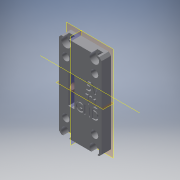
# Autodesk Inventor part: 02_Camera_Lid
Saved by Autodesk Inventor 2019.4 (Build 234330000, 330)
## iProperties
Created: 2021-09-23
Part Number: 02_Camera_Lid
Material: Generisch
Document SubType Name: Modeling
Designer: Muriel
Density: 1 g/cm^3
Appearance: Vorgabe
Author: Muriel
Autodesk Inventor part; units mm, degrees
ref_plane "YZ Plane" through (0, 0, 0) normal (1, 0, 0) x (0, 1, 0)
ref_plane "XZ Plane" through (0, 0, 0) normal (0, 1, 0) x (-1, 0, 0)
ref_plane "XY Plane" through (0, 0, 0) normal (0, 0, 1) x (1, 0, 0)
ref_plane "Arbeitsebene1" through (0, 0, 0) normal (0, 0, 1) x (1, 0, 0)
sketch "Skizze1" plane through (0, 0, 0) normal (0, 0, 1) x (1, 0, 0)
  line L0 (-3.05, 28.45) -> (-3.05, 27.95) projected
  line L1 (-2.75, 27.95) -> (-3.05, 27.95) projected
  line L2 (-1.75, 26.95) -> (-2.75, 27.95) projected
  line L3 (-1.75, 26.25) -> (-1.75, 26.95) projected
  line L4 (1.1, 26.25) -> (-1.75, 26.25) projected
  line L5 (1.1, 0.85) -> (1.1, 26.25) projected
  line L6 (1.1, 0.85) -> (-1.75, 0.85) projected
  line L7 (-1.75, 0.85) -> (-1.75, 0.15) projected
  line L8 (-2.75, -0.85) -> (-1.75, 0.15) projected
  line L9 (-2.75, -0.85) -> (-3.05, -0.85) projected
  line L10 (-3.05, -0.85) -> (-3.05, -1.35) projected
  line L11 (-3.05, -1.35) -> (-12.95, -1.35) projected
  line L12 (-12.95, -1.35) -> (-12.95, -0.35) projected
  line L13 (-12.95, -0.35) -> (-13.95, -0.35) projected
  line L14 (-13.95, -0.35) -> (-13.95, -1.35) projected
  line L15 (-13.95, -1.35) -> (-15.2198, -1.35) projected
  line L16 (-15.2198, -1.35) -> (-15.2198, 0.65) projected
  line L17 (-15.2198, 0.65) -> (-16.05, 0.65) projected
  line L18 (-16.05, 0.65) -> (-16.05, -3.35) projected
  line L19 (-15.05, -4.35) -> (-16.05, -3.35) projected
  line L20 (-15.05, -4.35) -> (0.75, -4.35) projected
  line L21 (1.75, -3.35) -> (0.75, -4.35) projected
  line L22 (1.75, -3.35) -> (1.75, 30.45) projected
  line L23 (0.75, 31.45) -> (1.75, 30.45) projected
  line L24 (-15.05, 31.45) -> (0.75, 31.45) projected
  line L25 (-16.05, 30.45) -> (-15.05, 31.45) projected
  line L26 (-16.05, 26.45) -> (-16.05, 30.45) projected
  line L27 (-16.05, 26.45) -> (-15.2198, 26.45) projected
  line L28 (-15.2198, 26.45) -> (-15.2198, 28.45) projected
  line L29 (-15.2198, 28.45) -> (-13.95, 28.45) projected
  line L30 (-13.95, 28.45) -> (-13.95, 27.45) projected
  line L31 (-13.95, 27.45) -> (-12.95, 27.45) projected
  line L32 (-12.95, 27.45) -> (-12.95, 28.45) projected
  line L33 (-12.95, 28.45) -> (-3.05, 28.45) projected
  circle A0 centre (-1.25, 29.85) radius 0.95 projected
  circle A1 centre (-13.05, 29.85) radius 0.95 projected
  circle A2 centre (-13.05, -2.75) radius 0.95 projected
  circle A3 centre (-1.25, -2.75) radius 0.95 projected
  line L34 (-16.05, 26.45) -> (-16.05, 0.65)
  point P0 (0, 0)
  constraints: 2 end point, 1 vertical
extrude "Extrusion1" add sketch "Skizze1" along normal blind 4
sketch "Skizze2" plane through (0, 0, 4) normal (0, 0, 1) x (1, 0, 0)
  circle A0 centre (-1.25, -2.75) radius 0.95 projected
  circle A1 centre (-13.05, -2.75) radius 0.95 projected
  circle A2 centre (-13.05, 29.85) radius 0.95 projected
  circle A3 centre (-1.25, 29.85) radius 0.95 projected
  line L0 (-16.05, 30.45) -> (-16.05, -3.35) projected
  line L1 (-16.05, -3.35) -> (-15.05, -4.35) projected
  line L2 (-15.05, -4.35) -> (0.75, -4.35) projected
  line L3 (0.75, -4.35) -> (1.75, -3.35) projected
  line L4 (1.75, -3.35) -> (1.75, 30.45) projected
  line L5 (1.75, 30.45) -> (0.75, 31.45) projected
  line L6 (0.75, 31.45) -> (-15.05, 31.45) projected
  line L7 (-15.05, 31.45) -> (-16.05, 30.45) projected
  point P0 (0, 0)
hole "Bohrung1" at (-1.25, 29.85, 4) at (-13.05, 29.85, 4) at (-1.25, -2.75, 4) at (-13.05, -2.75, 4) direction (0, 0, -1) diameter 2 depth 12 tip angle 118 counterbore diameter 4 counterbore depth 2.5
sketch "Skizze5" plane through (0, 0, 4) normal (0, 0, 1) x (1, 0, 0)
  line L0 (-5.0417, 20.4942) -> (0.4976, 20.4942) construction
  line L1 (0.4976, 20.4942) -> (0.4976, 16.9204) construction
  line L2 (0.4976, 16.9204) -> (-5.0417, 16.9204) construction
  line L3 (-5.0417, 16.9204) -> (-5.0417, 20.4942) construction
  line L4 (-9.0877, 11.2435) -> (0.5466, 11.2435) construction
  line L5 (0.5466, 11.2435) -> (0.5466, 7.613) construction
  line L6 (0.5466, 7.613) -> (-9.0877, 7.613) construction
  line L7 (-9.0877, 7.613) -> (-9.0877, 11.2435) construction
  line L8 (-5.1084, 15.6437) -> (0.3288, 15.6437) construction
  line L9 (0.3288, 15.6437) -> (0.3288, 12.1323) construction
  line L10 (0.3288, 12.1323) -> (-5.1084, 12.1323) construction
  line L11 (-5.1084, 12.1323) -> (-5.1084, 15.6437) construction
  spline S0 degree 2 poles (-2.6649, 18.106) (-2.6649, 17.8536) (-2.8266, 17.4225) (-2.9741, 17.2636) knots 0 0 0 1 2 2 2
  spline S1 degree 2 poles (-2.9741, 17.2636) (-3.1216, 17.1048) (-3.5612, 16.9204) (-3.8335, 16.9204) knots 0 0 0 1 2 2 2
  spline S2 degree 2 poles (-3.8335, 16.9204) (-4.0831, 16.9204) (-4.5709, 17.0311) (-4.7496, 17.119) knots 0 0 0 1 2 2 2
  line L12 (-4.7496, 17.119) -> (-4.7496, 17.6153)
  line L13 (-4.7496, 17.6153) -> (-4.7156, 17.6153)
  spline S3 degree 2 poles (-4.7156, 17.6153) (-4.6617, 17.5756) (-4.4603, 17.4735) (-4.3383, 17.4281) knots 0 0 0 1 2 2 2
  spline S4 degree 2 poles (-4.3383, 17.4281) (-4.1994, 17.3799) (-3.9696, 17.326) (-3.825, 17.326) knots 0 0 0 1 2 2 2
  spline S5 degree 2 poles (-3.825, 17.326) (-3.6831, 17.326) (-3.4165, 17.4281) (-3.3201, 17.5388) knots 0 0 0 1 2 2 2
  spline S6 degree 2 poles (-3.3201, 17.5388) (-3.2322, 17.6437) (-3.1414, 17.9217) (-3.1414, 18.1089) knots 0 0 0 1 2 2 2
  spline S7 degree 2 poles (-3.1414, 18.1089) (-3.1414, 18.2961) (-3.2435, 18.5343) (-3.34, 18.6137) knots 0 0 0 1 2 2 2
  spline S8 degree 2 poles (-3.34, 18.6137) (-3.4392, 18.7016) (-3.7342, 18.7754) (-3.9129, 18.7754) knots 0 0 0 1 2 2 2
  spline S9 degree 2 poles (-3.9129, 18.7754) (-4.1058, 18.7754) (-4.4887, 18.7158) (-4.6049, 18.6903) knots 0 0 0 1 2 2 2
  line L14 (-4.6049, 18.6903) -> (-4.6049, 20.4942)
  line L15 (-4.6049, 20.4942) -> (-2.6848, 20.4942)
  line L16 (-2.6848, 20.4942) -> (-2.6848, 20.0829)
  line L17 (-2.6848, 20.0829) -> (-4.154, 20.0829)
  line L18 (-4.154, 20.0829) -> (-4.154, 19.1498)
  spline S10 degree 2 poles (-4.154, 19.1498) (-4.0689, 19.1611) (-3.9044, 19.1696) (-3.8363, 19.1696) knots 0 0 0 1 2 2 2
  spline S11 degree 2 poles (-3.8363, 19.1696) (-3.5669, 19.1696) (-3.1953, 19.0817) (-3.0251, 18.9512) knots 0 0 0 1 2 2 2
  spline S12 degree 2 poles (-3.0251, 18.9512) (-2.8521, 18.8208) (-2.6649, 18.4237) (-2.6649, 18.106) knots 0 0 0 1 2 2 2
  line L19 (0.4777, 20.4942) -> (-0.7277, 16.9942)
  line L20 (-0.7277, 16.9942) -> (-1.2297, 16.9942)
  line L21 (-1.2297, 16.9942) -> (-2.4352, 20.4942)
  line L22 (-2.4352, 20.4942) -> (-1.936, 20.4942)
  line L23 (-1.936, 20.4942) -> (-0.966, 17.587)
  line L24 (-0.966, 17.587) -> (0.004, 20.4942)
  line L25 (0.004, 20.4942) -> (0.4777, 20.4942)
  line L26 (-3.937, 12.1323) -> (-3.937, 15.2182)
  line L27 (-3.937, 15.2182) -> (-5.1113, 15.2182)
  line L28 (-5.1113, 15.2182) -> (-5.1113, 15.6323)
  line L29 (-5.1113, 15.6323) -> (-2.2976, 15.6323)
  line L30 (-2.2976, 15.6323) -> (-2.2976, 15.2182)
  line L31 (-2.2976, 15.2182) -> (-3.4719, 15.2182)
  line L32 (-3.4719, 15.2182) -> (-3.4719, 12.1323)
  line L33 (-3.4719, 12.1323) -> (-3.937, 12.1323)
  line L34 (-0.0598, 12.1323) -> (-1.7673, 12.1323)
  line L35 (-1.7673, 12.1323) -> (-1.7673, 12.4897)
  line L36 (-1.7673, 12.4897) -> (-1.1319, 12.4897)
  line L37 (-1.1319, 12.4897) -> (-1.1319, 14.8353)
  line L38 (-1.1319, 14.8353) -> (-1.7673, 14.8353)
  line L39 (-1.7673, 14.8353) -> (-1.7673, 15.1558)
  spline S13 degree 2 poles (-1.7673, 15.1558) (-1.407, 15.1558) (-1.0667, 15.36) (-1.044, 15.6437) knots 0 0 0 1 2 2 2
  line L40 (-1.044, 15.6437) -> (-0.6809, 15.6437)
  line L41 (-0.6809, 15.6437) -> (-0.6809, 12.4897)
  line L42 (-0.6809, 12.4897) -> (-0.0598, 12.4897)
  line L43 (-0.0598, 12.4897) -> (-0.0598, 12.1323)
  spline S14 degree 2 poles (-7.2668, 7.613) (-7.6384, 7.613) (-8.2538, 7.8399) (-8.4751, 8.0696) knots 0 0 0 1 2 2 2
  spline S15 degree 2 poles (-8.4751, 8.0696) (-8.6963, 8.3022) (-8.9317, 8.9886) (-8.9317, 9.4339) knots 0 0 0 1 2 2 2
  spline S16 degree 2 poles (-8.9317, 9.4339) (-8.9317, 9.8565) (-8.6935, 10.5259) (-8.4722, 10.7641) knots 0 0 0 1 2 2 2
  spline S17 degree 2 poles (-8.4722, 10.7641) (-8.2595, 10.9939) (-7.6355, 11.2435) (-7.264, 11.2435) knots 0 0 0 1 2 2 2
  spline S18 degree 2 poles (-7.264, 11.2435) (-7.0853, 11.2435) (-6.7619, 11.1924) (-6.6144, 11.147) knots 0 0 0 1 2 2 2
  spline S19 degree 2 poles (-6.6144, 11.147) (-6.4953, 11.113) (-6.206, 10.9882) (-6.1181, 10.9428) knots 0 0 0 1 2 2 2
  line L44 (-6.1181, 10.9428) -> (-6.1181, 10.3812)
  line L45 (-6.1181, 10.3812) -> (-6.1578, 10.3812)
  spline S20 degree 2 poles (-6.1578, 10.3812) (-6.2457, 10.4578) (-6.4301, 10.5968) (-6.6003, 10.6762) knots 0 0 0 1 2 2 2
  spline S21 degree 2 poles (-6.6003, 10.6762) (-6.7421, 10.7471) (-7.108, 10.8407) (-7.3179, 10.8407) knots 0 0 0 1 2 2 2
  spline S22 degree 2 poles (-7.3179, 10.8407) (-7.8227, 10.8407) (-8.4467, 10.0806) (-8.4467, 9.4481) knots 0 0 0 1 2 2 2
  spline S23 degree 2 poles (-8.4467, 9.4481) (-8.4467, 9.0964) (-8.2822, 8.5688) (-8.1262, 8.3873) knots 0 0 0 1 2 2 2
  spline S24 degree 2 poles (-8.1262, 8.3873) (-7.9759, 8.2058) (-7.5504, 8.0157) (-7.2838, 8.0157) knots 0 0 0 1 2 2 2
  spline S25 degree 2 poles (-7.2838, 8.0157) (-7.0881, 8.0157) (-6.6967, 8.0725) (-6.5634, 8.1292) knots 0 0 0 1 2 2 2
  line L46 (-6.5634, 8.1292) -> (-6.5634, 9.034)
  line L47 (-6.5634, 9.034) -> (-7.3746, 9.034)
  line L48 (-7.3746, 9.034) -> (-7.3746, 9.4424)
  line L49 (-7.3746, 9.4424) -> (-6.1039, 9.4424)
  line L50 (-6.1039, 9.4424) -> (-6.1039, 7.9136)
  spline S26 degree 2 poles (-6.1039, 7.9136) (-6.1918, 7.8739) (-6.4925, 7.752) (-6.6201, 7.7151) knots 0 0 0 1 2 2 2
  spline S27 degree 2 poles (-6.6201, 7.7151) (-6.7931, 7.664) (-7.0711, 7.613) (-7.2668, 7.613) knots 0 0 0 1 2 2 2
  line L51 (-3.0152, 7.6811) -> (-3.5371, 7.6811)
  line L52 (-3.5371, 7.6811) -> (-5.0857, 10.6989)
  line L53 (-5.0857, 10.6989) -> (-5.0857, 7.6811)
  line L54 (-5.0857, 7.6811) -> (-5.5196, 7.6811)
  line L55 (-5.5196, 7.6811) -> (-5.5196, 11.1811)
  line L56 (-5.5196, 11.1811) -> (-4.8588, 11.1811)
  line L57 (-4.8588, 11.1811) -> (-3.4491, 8.41)
  line L58 (-3.4491, 8.41) -> (-3.4491, 11.1811)
  line L59 (-3.4491, 11.1811) -> (-3.0152, 11.1811)
  line L60 (-3.0152, 11.1811) -> (-3.0152, 7.6811)
  spline S28 degree 2 poles (0.4536, 9.4282) (0.4536, 8.9489) (0.065, 8.1774) (-0.2611, 7.9619) knots 0 0 0 1 2 2 2
  spline S29 degree 2 poles (-0.2611, 7.9619) (-0.5277, 7.7945) (-1.0751, 7.6811) (-1.5006, 7.6811) knots 0 0 0 1 2 2 2
  line L61 (-1.5006, 7.6811) -> (-2.3061, 7.6811)
  line L62 (-2.3061, 7.6811) -> (-2.3061, 11.1811)
  line L63 (-2.3061, 11.1811) -> (-1.5091, 11.1811)
  spline S30 degree 2 poles (-1.5091, 11.1811) (-1.0156, 11.1811) (-0.454, 11.0336) (-0.2555, 10.9031) knots 0 0 0 1 2 2 2
  spline S31 degree 2 poles (-0.2555, 10.9031) (0.0821, 10.679) (0.4536, 9.9388) (0.4536, 9.4282) knots 0 0 0 1 2 2 2
  spline S32 degree 2 poles (-0.0314, 9.4339) (-0.0314, 9.8367) (-0.298, 10.4068) (-0.5618, 10.5684) knots 0 0 0 1 2 2 2
  spline S33 degree 2 poles (-0.5618, 10.5684) (-0.749, 10.679) (-1.1716, 10.7783) (-1.4864, 10.7783) knots 0 0 0 1 2 2 2
  line L64 (-1.4864, 10.7783) -> (-1.8409, 10.7783)
  line L65 (-1.8409, 10.7783) -> (-1.8409, 8.0838)
  line L66 (-1.8409, 8.0838) -> (-1.4864, 8.0838)
  spline S34 degree 2 poles (-1.4864, 8.0838) (-1.1773, 8.0838) (-0.7093, 8.1831) (-0.5192, 8.3164) knots 0 0 0 1 2 2 2
  spline S35 degree 2 poles (-0.5192, 8.3164) (-0.2753, 8.4809) (-0.0314, 9.0255) (-0.0314, 9.4339) knots 0 0 0 1 2 2 2
  point P0 (0, 0)
  constraints: 6 other
extrude "Extrusion3" cut sketch "Skizze5" against normal blind 1
sketch "Skizze6" plane through (0, 0, 4) normal (0, 0, 1) x (1, 0, 0)
  arc A0 (-0.05, -4.35) -> (-2.45, -4.35) centre (-1.25, -2.75) ccw projected
  line L0 (-0.05, -4.35) -> (0.75, -4.35) projected
  line L1 (0.75, -4.35) -> (1.75, -3.35) projected
  line L2 (1.75, -3.35) -> (1.75, 30.45) projected
  line L3 (1.75, 30.45) -> (0.75, 31.45) projected
  line L4 (0.75, 31.45) -> (-0.05, 31.45) projected
  arc A1 (-2.45, 31.45) -> (-0.05, 31.45) centre (-1.25, 29.85) ccw projected
  line L5 (-2.45, 31.45) -> (-11.85, 31.45) projected
  arc A2 (-14.25, 31.45) -> (-11.85, 31.45) centre (-13.05, 29.85) ccw projected
  line L6 (-14.25, 31.45) -> (-15.05, 31.45) projected
  line L7 (-15.05, 31.45) -> (-16.05, 30.45) projected
  line L8 (-16.05, 30.45) -> (-16.05, -3.35) projected
  line L9 (-16.05, -3.35) -> (-15.05, -4.35) projected
  line L10 (-15.05, -4.35) -> (-14.25, -4.35) projected
  arc A3 (-11.85, -4.35) -> (-14.25, -4.35) centre (-13.05, -2.75) ccw projected
  line L11 (-11.85, -4.35) -> (-2.45, -4.35) projected
  line L12 (-3.0152, 11.1811) -> (-3.0152, 7.6811) projected
  line L13 (-3.0152, 7.6811) -> (-3.5371, 7.6811) projected
  line L14 (-3.5371, 7.6811) -> (-5.0857, 10.6989) projected
  line L15 (-5.0857, 10.6989) -> (-5.0857, 7.6811) projected
  line L16 (-5.0857, 7.6811) -> (-5.5196, 7.6811) projected
  line L17 (-5.5196, 7.6811) -> (-5.5196, 11.1811) projected
  line L18 (-5.5196, 11.1811) -> (-4.8588, 11.1811) projected
  line L19 (-4.8588, 11.1811) -> (-3.4491, 8.41) projected
  line L20 (-3.4491, 8.41) -> (-3.4491, 11.1811) projected
  line L21 (-3.4491, 11.1811) -> (-3.0152, 11.1811) projected
  line L22 (-0.0598, 12.4897) -> (-0.0598, 12.1323) projected
  line L23 (-0.0598, 12.1323) -> (-1.7673, 12.1323) projected
  line L24 (-1.7673, 12.1323) -> (-1.7673, 12.4897) projected
  line L25 (-1.7673, 12.4897) -> (-1.1319, 12.4897) projected
  line L26 (-1.1319, 12.4897) -> (-1.1319, 14.8353) projected
  line L27 (-1.1319, 14.8353) -> (-1.7673, 14.8353) projected
  line L28 (-1.7673, 14.8353) -> (-1.7673, 15.1558) projected
  line L29 (-1.044, 15.6437) -> (-0.6809, 15.6437) projected
  line L30 (-0.6809, 15.6437) -> (-0.6809, 12.4897) projected
  line L31 (-0.6809, 12.4897) -> (-0.0598, 12.4897) projected
  line L32 (0.004, 20.4942) -> (0.4777, 20.4942) projected
  line L33 (0.4777, 20.4942) -> (-0.7277, 16.9942) projected
  line L34 (-0.7277, 16.9942) -> (-1.2297, 16.9942) projected
  line L35 (-1.2297, 16.9942) -> (-2.4352, 20.4942) projected
  line L36 (-2.4352, 20.4942) -> (-1.936, 20.4942) projected
  line L37 (-1.936, 20.4942) -> (-0.966, 17.587) projected
  line L38 (-0.966, 17.587) -> (0.004, 20.4942) projected
  line L39 (-4.7496, 17.119) -> (-4.7496, 17.6153) projected
  line L40 (-4.7496, 17.6153) -> (-4.7156, 17.6153) projected
  line L41 (-4.6049, 18.6903) -> (-4.6049, 20.4942) projected
  line L42 (-4.6049, 20.4942) -> (-2.6848, 20.4942) projected
  line L43 (-2.6848, 20.4942) -> (-2.6848, 20.0829) projected
  line L44 (-2.6848, 20.0829) -> (-4.154, 20.0829) projected
  line L45 (-4.154, 20.0829) -> (-4.154, 19.1498) projected
  line L46 (-3.4719, 12.1323) -> (-3.937, 12.1323) projected
  line L47 (-3.937, 12.1323) -> (-3.937, 15.2182) projected
  line L48 (-3.937, 15.2182) -> (-5.1113, 15.2182) projected
  line L49 (-5.1113, 15.2182) -> (-5.1113, 15.6323) projected
  line L50 (-5.1113, 15.6323) -> (-2.2976, 15.6323) projected
  line L51 (-2.2976, 15.6323) -> (-2.2976, 15.2182) projected
  line L52 (-2.2976, 15.2182) -> (-3.4719, 15.2182) projected
  line L53 (-3.4719, 15.2182) -> (-3.4719, 12.1323) projected
  line L54 (-6.1181, 10.9428) -> (-6.1181, 10.3812) projected
  line L55 (-6.1181, 10.3812) -> (-6.1578, 10.3812) projected
  line L56 (-6.5634, 8.1292) -> (-6.5634, 9.034) projected
  line L57 (-6.5634, 9.034) -> (-7.3746, 9.034) projected
  line L58 (-7.3746, 9.034) -> (-7.3746, 9.4424) projected
  line L59 (-7.3746, 9.4424) -> (-6.1039, 9.4424) projected
  line L60 (-6.1039, 9.4424) -> (-6.1039, 7.9136) projected
  line L61 (-1.5006, 7.6811) -> (-2.3061, 7.6811) projected
  line L62 (-2.3061, 7.6811) -> (-2.3061, 11.1811) projected
  line L63 (-2.3061, 11.1811) -> (-1.5091, 11.1811) projected
  line L64 (-9.6163, 19.7) -> (-9.6163, 7.4)
  line L65 (-9.6163, 7.4) -> (-12.1163, 7.4)
  line L66 (-12.1163, 7.4) -> (-12.1163, 19.7)
  line L67 (-12.1163, 19.7) -> (-9.6163, 19.7)
  line L68 (-9.6163, 19.7) -> (-12.1163, 7.4) construction
  line L69 (-9.6163, 7.4) -> (-12.1163, 19.7) construction
  point P0 (0, 0)
  point P1 (-10.8663, 13.55)
  dimension "d31" = 12.3
  dimension "d32" = 2.5
  dimension "d38" = 17.9
  constraints: 12 end point, 2 midpoint, 2 parallel, 1 perpendicular, 1 vertical, 32 other
  measures "d31" distance of L64.start L64.end
  measures "d32" distance of L64.end L65.end
  measures "d38" distance from line of point (-10.866, 13.55) L11
extrude "Extrusion4" cut sketch "Skizze6" against normal blind 10 contours L64 L65 L66 L67
sketch "Skizze7" plane through (-16.05, -3.35, 0) normal (-1, 0, 0) x (0, 0, 1)
  line L0 (0, 33.8) -> (0, 0) projected
  line L1 (0, 0) -> (4, 0) projected
  line L2 (4, 33.8) -> (4, 0) projected
  line L3 (0, 33.8) -> (4, 33.8) projected
  circle A0 centre (2, 16.9) radius 1.4
  point P0 (0, 3.35)
  dimension "d35" = 2.8
  constraints: 1 centre point
  measures "d35" diameter of A0
extrude "Extrusion5" cut sketch "Skizze7" against normal up to next contours A0
sketch "Skizze8" plane through (0, 0, 4) normal (0, 0, 1) x (1, 0, 0)
  line L0 (-12.1163, 19.7) -> (-9.6163, 19.7) projected
  line L1 (-9.6163, 19.7) -> (-9.6163, 7.4) projected
  line L2 (-9.6163, 7.4) -> (-12.1163, 7.4) projected
  line L3 (-12.1163, 7.4) -> (-12.1163, 19.7) projected
  arc A0 (-0.05, -4.35) -> (-2.45, -4.35) centre (-1.25, -2.75) ccw projected
  line L4 (-0.05, -4.35) -> (0.75, -4.35) projected
  line L5 (0.75, -4.35) -> (1.75, -3.35) projected
  line L6 (1.75, -3.35) -> (1.75, 30.45) projected
  line L7 (1.75, 30.45) -> (0.75, 31.45) projected
  line L8 (0.75, 31.45) -> (-0.05, 31.45) projected
  arc A1 (-2.45, 31.45) -> (-0.05, 31.45) centre (-1.25, 29.85) ccw projected
  line L9 (-2.45, 31.45) -> (-11.85, 31.45) projected
  arc A2 (-14.25, 31.45) -> (-11.85, 31.45) centre (-13.05, 29.85) ccw projected
  line L10 (-14.25, 31.45) -> (-15.05, 31.45) projected
  line L11 (-15.05, 31.45) -> (-16.05, 30.45) projected
  line L12 (-16.05, 30.45) -> (-16.05, -3.35) projected
  line L13 (-16.05, -3.35) -> (-15.05, -4.35) projected
  line L14 (-15.05, -4.35) -> (-14.25, -4.35) projected
  arc A3 (-11.85, -4.35) -> (-14.25, -4.35) centre (-13.05, -2.75) ccw projected
  line L15 (-11.85, -4.35) -> (-2.45, -4.35) projected
  line L16 (-3.0152, 11.1811) -> (-3.0152, 7.6811) projected
  line L17 (-3.0152, 7.6811) -> (-3.5371, 7.6811) projected
  line L18 (-3.5371, 7.6811) -> (-5.0857, 10.6989) projected
  line L19 (-5.0857, 10.6989) -> (-5.0857, 7.6811) projected
  line L20 (-5.0857, 7.6811) -> (-5.5196, 7.6811) projected
  line L21 (-5.5196, 7.6811) -> (-5.5196, 11.1811) projected
  line L22 (-5.5196, 11.1811) -> (-4.8588, 11.1811) projected
  line L23 (-4.8588, 11.1811) -> (-3.4491, 8.41) projected
  line L24 (-3.4491, 8.41) -> (-3.4491, 11.1811) projected
  line L25 (-3.4491, 11.1811) -> (-3.0152, 11.1811) projected
  line L26 (-0.0598, 12.4897) -> (-0.0598, 12.1323) projected
  line L27 (-0.0598, 12.1323) -> (-1.7673, 12.1323) projected
  line L28 (-1.7673, 12.1323) -> (-1.7673, 12.4897) projected
  line L29 (-1.7673, 12.4897) -> (-1.1319, 12.4897) projected
  line L30 (-1.1319, 12.4897) -> (-1.1319, 14.8353) projected
  line L31 (-1.1319, 14.8353) -> (-1.7673, 14.8353) projected
  line L32 (-1.7673, 14.8353) -> (-1.7673, 15.1558) projected
  line L33 (-1.044, 15.6437) -> (-0.6809, 15.6437) projected
  line L34 (-0.6809, 15.6437) -> (-0.6809, 12.4897) projected
  line L35 (-0.6809, 12.4897) -> (-0.0598, 12.4897) projected
  line L36 (0.004, 20.4942) -> (0.4777, 20.4942) projected
  line L37 (0.4777, 20.4942) -> (-0.7277, 16.9942) projected
  line L38 (-0.7277, 16.9942) -> (-1.2297, 16.9942) projected
  line L39 (-1.2297, 16.9942) -> (-2.4352, 20.4942) projected
  line L40 (-2.4352, 20.4942) -> (-1.936, 20.4942) projected
  line L41 (-1.936, 20.4942) -> (-0.966, 17.587) projected
  line L42 (-0.966, 17.587) -> (0.004, 20.4942) projected
  line L43 (-4.7496, 17.119) -> (-4.7496, 17.6153) projected
  line L44 (-4.7496, 17.6153) -> (-4.7156, 17.6153) projected
  line L45 (-4.6049, 18.6903) -> (-4.6049, 20.4942) projected
  line L46 (-4.6049, 20.4942) -> (-2.6848, 20.4942) projected
  line L47 (-2.6848, 20.4942) -> (-2.6848, 20.0829) projected
  line L48 (-2.6848, 20.0829) -> (-4.154, 20.0829) projected
  line L49 (-4.154, 20.0829) -> (-4.154, 19.1498) projected
  line L50 (-3.4719, 12.1323) -> (-3.937, 12.1323) projected
  line L51 (-3.937, 12.1323) -> (-3.937, 15.2182) projected
  line L52 (-3.937, 15.2182) -> (-5.1113, 15.2182) projected
  line L53 (-5.1113, 15.2182) -> (-5.1113, 15.6323) projected
  line L54 (-5.1113, 15.6323) -> (-2.2976, 15.6323) projected
  line L55 (-2.2976, 15.6323) -> (-2.2976, 15.2182) projected
  line L56 (-2.2976, 15.2182) -> (-3.4719, 15.2182) projected
  line L57 (-3.4719, 15.2182) -> (-3.4719, 12.1323) projected
  line L58 (-6.1181, 10.9428) -> (-6.1181, 10.3812) projected
  line L59 (-6.1181, 10.3812) -> (-6.1578, 10.3812) projected
  line L60 (-6.5634, 8.1292) -> (-6.5634, 9.034) projected
  line L61 (-6.5634, 9.034) -> (-7.3746, 9.034) projected
  line L62 (-7.3746, 9.034) -> (-7.3746, 9.4424) projected
  line L63 (-7.3746, 9.4424) -> (-6.1039, 9.4424) projected
  line L64 (-6.1039, 9.4424) -> (-6.1039, 7.9136) projected
  line L65 (-1.5006, 7.6811) -> (-2.3061, 7.6811) projected
  line L66 (-2.3061, 7.6811) -> (-2.3061, 11.1811) projected
  line L67 (-2.3061, 11.1811) -> (-1.5091, 11.1811) projected
  line L68 (-1.15, 24.55) -> (-13.15, 24.55) construction
  line L69 (-13.15, 24.55) -> (-13.15, 2.55) construction
  line L70 (-13.15, 2.55) -> (-1.15, 2.55) construction
  line L71 (-1.15, 2.55) -> (-1.15, 24.55) construction
  line L72 (-1.15, 24.55) -> (-13.15, 2.55) construction
  line L73 (-13.15, 24.55) -> (-1.15, 2.55) construction
  circle A4 centre (-13.15, 2.55) radius 1.5
  circle A5 centre (-13.15, 24.55) radius 1.5
  circle A6 centre (-1.15, 24.55) radius 1.5
  circle A7 centre (-1.15, 2.55) radius 1.5
  point P0 (0, 0)
  point P1 (-7.15, 13.55)
  dimension "d39" = 12
  dimension "d40" = 22
  dimension "d41" = 17.9
  dimension "d42" = 8.9
  dimension "d43" = 3
  dimension "d44" = 3
  dimension "d45" = 3
  dimension "d46" = 3
  constraints: 12 end point, 4 centre point, 4 coincident, 2 midpoint, 2 parallel, 1 horizontal, 1 perpendicular, 32 other
  measures "d39" distance of L70.end L69.end
  measures "d40" distance of L69.end L68.end
  measures "d41" distance from line of point (-7.15, 13.55) L15
  measures "d42" distance from line of point (-7.15, 13.55) L12
  measures "d43" diameter of A4
  measures "d44" diameter of A5
  measures "d45" diameter of A6
  measures "d46" diameter of A7
extrude "Extrusion6" cut sketch "Skizze8" against normal blind 3 draft -4 contours A4 | A5 | A6 | A7
sketch "Skizze9" plane through (0, 0, 0) normal (0, 0, -1) x (-1, 0, 0)
  line L0 (12.1163, 19.7) -> (12.1163, 7.4) projected
  line L1 (9.6163, 7.4) -> (9.6163, 19.7) projected
  line L2 (12.1163, 7.4) -> (9.6163, 7.4) projected
  line L3 (9.6163, 19.7) -> (12.1163, 19.7) projected
  line L4 (9.6163, 19.7) -> (12.1163, 19.7) projected
  line L5 (12.1163, 19.7) -> (12.1163, 7.4) projected
  line L6 (12.1163, 7.4) -> (9.6163, 7.4) projected
  line L7 (9.6163, 7.4) -> (9.6163, 19.7) projected
  circle A0 centre (1.25, -2.75) radius 1 projected
  circle A1 centre (1.25, 29.85) radius 1 projected
  circle A2 centre (13.05, 29.85) radius 1 projected
  circle A3 centre (13.05, -2.75) radius 1 projected
  line L8 (16.05, 30.45) -> (16.05, -3.35) projected
  line L9 (15.05, 31.45) -> (16.05, 30.45) projected
  line L10 (-0.75, 31.45) -> (15.05, 31.45) projected
  line L11 (-1.75, 30.45) -> (-0.75, 31.45) projected
  line L12 (-1.75, -3.35) -> (-1.75, 30.45) projected
  line L13 (-0.75, -4.35) -> (-1.75, -3.35) projected
  line L14 (15.05, -4.35) -> (-0.75, -4.35) projected
  line L15 (16.05, -3.35) -> (15.05, -4.35) projected
  line L16 (10.0163, 19.3) -> (10.0163, 7.8)
  line L17 (10.0163, 7.8) -> (11.7163, 7.8)
  line L18 (11.7163, 7.8) -> (11.7163, 19.3)
  line L19 (11.7163, 19.3) -> (10.0163, 19.3)
  point P0 (0, 0)
  dimension "d49" = 0.4
  constraints: 8 end point, 3 other
  measures "d49" distance between parallel lines of L1 L16
extrude "Extrusion7" add sketch "Skizze9" against normal blind 1 contours L0 L2 L1 L3
ref_plane "Work Plane2" through (0, 19.7, 4) normal (0, -0.7071068, 0.7071068) x (1, 0, 0)
ref_plane "Work Plane3" through (-12.1163, 13.55, 4) normal (0, 1, 0) x (1, 0, 0)
ref_plane "Work Plane4" through (-10.8663, 7.4, 4) normal (-1, 0, 0) x (0, 0, 1)
